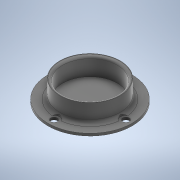
# Autodesk Inventor part: Chute
Saved by Autodesk Inventor 2020.2 (Build 242310000, 310)
## iProperties
Created: 2020-10-16
Part Number: Chute
Material: Generic
Document SubType Name: Modeling
Designer: JK
Density: 1 g/cm^3
Appearance: Smooth - Black
Author: JK
Autodesk Inventor part; units mm, degrees
ref_plane "YZ Plane" through (0, 0, 0) normal (1, 0, 0) x (0, 1, 0)
ref_plane "XZ Plane" through (0, 0, 0) normal (0, 1, 0) x (-1, 0, 0)
ref_plane "XY Plane" through (0, 0, 0) normal (0, 0, 1) x (1, 0, 0)
sketch "Sketch9" plane through (0, 0, 0) normal (0, 1, 0) x (-1, 0, 0)
  circle A0 centre (0, 0) radius 22.8
  circle A1 centre (0, 0) radius 25.2
  dimension "d31" = 45.6
  dimension "d32" = 2.4
  constraints: 2 centre point, 2 coincident
  measures "d31" diameter of A0
  measures "d32" radial gap between concentric circles of A1 A0
extrude "Extrusion7" add sketch "Sketch9" along normal blind 15
sketch "Sketch10" plane through (0, 0, 0) normal (0, -1, 0) x (1, 0, 0)
  circle A0 centre (0, 0) radius 25.2
  constraints: 1 centre point, 1 coincident
extrude "Extrusion8" add sketch "Sketch10" along normal blind 2
sketch "Sketch11" plane through (0, -2, 0) normal (0, -1, 0) x (1, 0, 0)
  circle A0 centre (0, 0) radius 35
  circle A1 centre (0, 30) radius 2.75
  circle A2 centre (0, -30) radius 2.75
  circle A3 centre (30, 0) radius 2.75
  circle A4 centre (-30, 0) radius 2.75
  dimension "d37" = 60
  dimension "d38" = 5.5
  dimension "d39" = 5.5
  dimension "d40" = 30
  dimension "d41" = 70
  dimension "d42" = 30
  dimension "d43" = 60
  constraints: 5 centre point, 2 equal radius, 1 coincident, 1 horizontal alignment, 1 vertical alignment
  measures "d37" distance of A2.centre A1.centre
  measures "d38" diameter of A1
  measures "d39" diameter of A2
  measures "d40" distance of A1.centre point (0, 0)
  measures "d41" diameter of A0
  measures "d42" distance of A3.centre point (0, 0)
  measures "d43" distance of A3.centre A4.centre
extrude "Extrusion9" add sketch "Sketch11" against normal blind 2
fillet "Fillet2" radius 2 1 edges at (22.8, 15, 0)
fillet "Fillet3" radius 3 1 edges at (25.2, 0, 0)
sketch "Sketch12" plane through (0, 0, 0) normal (0, 1, 0) x (1, 0, 0)
  circle A0 centre (0, -30) radius 2.75 projected
  circle A1 centre (0, -30) radius 4.5
  point P0 (0, 0)
  dimension "d48" = 9
  constraints: 1 centre point, 1 coincident
  measures "d48" diameter of A1
extrude "Extrusion10" cut sketch "Sketch12" along normal blind 10 contours A0 | A1
pattern_circular "Circular Pattern1" count 4 over 360 about axis through (0, 0, 0) along (0, 1, 0) of "Extrusion10"
body "Solid2"
